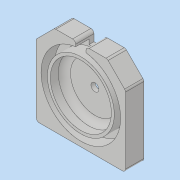
# Autodesk Inventor part: BallastTankMillFixture
Saved by Autodesk Inventor 2017.3 (Build 213256000, 256)
## iProperties
Created: 2018-07-14
Part Number: BallastTankMillFixture
Material: Generic
Document SubType Name: Modeling
Designer: Derek Wider
Density: 1 g/cm^3
Appearance: Default
Author: Derek Wider
Autodesk Inventor part; units mm, degrees
ref_plane "YZ Plane" through (0, 0, 0) normal (1, 0, 0) x (0, 1, 0)
ref_plane "XZ Plane" through (0, 0, 0) normal (0, 1, 0) x (-1, 0, 0)
ref_plane "XY Plane" through (0, 0, 0) normal (0, 0, 1) x (1, 0, 0)
sketch "Sketch1" plane through (0, 0, 0) normal (0, 0, 1) x (1, 0, 0)
  circle A0 centre (0, 0) radius 31.75
  circle A1 centre (0, 0) radius 34.798
  circle A2 centre (0, 0) radius 41.402
  line L0 (-46.482, 46.482) -> (46.482, 46.482)
  line L1 (46.482, 46.482) -> (46.482, -46.482)
  line L2 (46.482, -46.482) -> (-46.482, -46.482)
  line L3 (-46.482, -46.482) -> (-46.482, 46.482)
  line L4 (0, 46.482) -> (0, 41.402) construction
  line L5 (0, -41.402) -> (0, -46.482) construction
  line L6 (-46.482, 0) -> (-41.402, 0) construction
  line L7 (46.482, 0) -> (41.402, 0) construction
  dimension "d0" = 63.5
  dimension "d1" = 69.596
  dimension "d2" = 82.804
  dimension "d3" = 5.08
  constraints: 16 end point, 4 midpoint, 4 perpendicular, 4 point on circle, 3 centre point, 3 coincident, 3 horizontal, 2 parallel, 2 vertical
  measures "d0" diameter of A0
  measures "d1" diameter of A1
  measures "d2" diameter of A2
  measures "d3" distance of L4.start L4.end
extrude "Extrusion1" add sketch "Sketch1" along normal blind 5.08 contours A1 | A2 | L0 L1 L2 L3
extrude "Extrusion2" add sketch "Sketch1" along normal blind 19.05 contours A1
extrude "Extrusion3" add sketch "Sketch1" along normal blind 19.05 contours L0 L1 L2 L3
sketch "Sketch2" plane through (0, 0, 0) normal (0, 0, -1) x (-1, 0, 0)
  circle A0 centre (0, 0) radius 34.798 construction
  line L0 (46.482, 46.482) -> (-46.482, 46.482) projected
  line L1 (-5.3975, 46.482) -> (5.3975, 46.482)
  line L2 (5.3975, 46.482) -> (5.3975, 36.068)
  line L3 (5.3975, 36.068) -> (-5.3975, 36.068)
  line L4 (-5.3975, 36.068) -> (-5.3975, 46.482)
  line L5 (0, 34.798) -> (0, 36.068) construction
  dimension "d10" = 10.795
  dimension "d11" = 1.27
  constraints: 10 end point, 2 parallel, 2 perpendicular, 2 vertical alignment, 1 horizontal, 1 midpoint, 1 point on line, 1 other
  measures "d10" distance between parallel lines of L4 L2
  measures "d11" distance of L5.start L5.end
extrude "Extrusion4" cut sketch "Sketch2" against normal blind 19.05
chamfer "Chamfer1" distance 19.05 angle 45 2 edges at (46.482, 46.482, 9.525) (-46.482, 46.482, 9.525)
fillet "Fillet1" radius 3.175 8 edges at (46.482, -46.482, 9.525) (46.482, 27.432, 9.525) (27.432, 46.482, 9.525) (5.3975, 46.482, 9.525) (-5.3975, 46.482, 9.525) (-27.432, 46.482, 9.525) (-46.482, 27.432, 9.525) (-46.482, -46.482, 9.525)
sketch "Sketch3" plane through (0, 0, 0) normal (0, 0, -1) x (-1, 0, 0)
  circle A0 centre (0, 0) radius 31.75 projected
  circle A1 centre (0, 0) radius 4.1275
  dimension "d18" = 8.255
  constraints: 1 centre point, 1 coincident
  measures "d18" diameter of A1
extrude "Extrusion5" add sketch "Sketch3" against normal blind 4.445
fillet "Fillet2" radius 6.35 1 edges at (-31.75, 0, 4.445)
body "Solid1"
